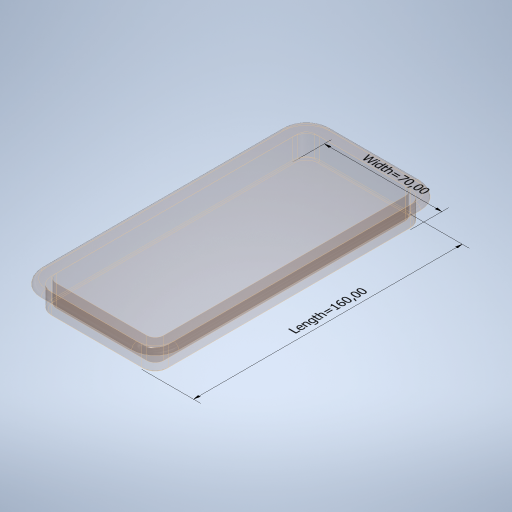
# Autodesk Inventor part: Holder for paper clips-01
Saved by Autodesk Inventor 2024 (Build 280153000, 153)
## iProperties
Company: UAB Čeli APS
Created: 2022-04-25
Part Number: Holder for paper clips-01
Material: Polycarbonate, Smoke
Document SubType Name: Modeling
Designer: sauliusd
Density: 1.2 g/cm^3
Appearance: Polycarbonate - Smoked
Description: Holder for paper clips.ipt
Width: 70,000 mm
Length: 160,000 mm
Author: S. Dereškevičius
Autodesk Inventor part; units mm, degrees
ref_plane "YZ Plane" through (0, 0, 0) normal (1, 0, 0) x (0, 1, 0)
ref_plane "XZ Plane" through (0, 0, 0) normal (0, 1, 0) x (-1, 0, 0)
ref_plane "XY Plane" through (0, 0, 0) normal (0, 0, 1) x (1, 0, 0)
sketch "Sketch1" plane through (0, 0, 0) normal (0, 0, 1) x (1, 0, 0)
  line L0 (-80, -35) -> (80, -35)
  line L1 (80, -35) -> (80, 35)
  line L2 (80, 35) -> (-80, 35)
  line L3 (-80, 35) -> (-80, -35)
  line L4 (-80, -35) -> (80, 35) construction
  line L5 (80, -35) -> (-80, 35) construction
  point P0 (0, 0)
  constraints: 12 end point, 2 midpoint, 2 parallel, 1 horizontal, 1 horizontal alignment, 1 perpendicular, 1 vertical alignment
extrude "Extrusion1" add sketch "Sketch1" along normal blind 13
fillet "Fillet1" radius 8 4 edges at (-80, -35, 6.5) (-80, 35, 6.5) (80, -35, 6.5) (80, 35, 6.5)
shell "Shell1" thickness 3 removed faces 1 at (24, -11.6667, 13)
sketch "Sketch2" plane through (0, 0, 13) normal (0, 0, 1) x (1, 0, 0)
  arc A0 (80, 27) -> (72, 35) centre (72, 27) ccw projected
  line L0 (72, 35) -> (-72, 35) projected
  arc A1 (-72, 35) -> (-80, 27) centre (-72, 27) ccw projected
  line L1 (-80, 27) -> (-80, -27) projected
  arc A2 (-80, -27) -> (-72, -35) centre (-72, -27) ccw projected
  line L2 (-72, -35) -> (72, -35) projected
  arc A3 (72, -35) -> (80, -27) centre (72, -27) ccw projected
  line L3 (80, -27) -> (80, 27) projected
  line L4 (-72, 41) -> (72, 41)
  arc A4 (86, 27) -> (72, 41) centre (72, 27) ccw
  line L5 (86, 27) -> (86, -27)
  arc A5 (72, -41) -> (86, -27) centre (72, -27) ccw
  line L6 (72, -41) -> (-72, -41)
  arc A6 (-86, -27) -> (-72, -41) centre (-72, -27) ccw
  line L7 (-86, -27) -> (-86, 27)
  arc A7 (-72, 41) -> (-86, 27) centre (-72, 27) ccw
  arc A8 (-72, 32) -> (-77, 27) centre (-72, 27) ccw projected
  line L8 (-72, 32) -> (72, 32) projected
  arc A9 (77, 27) -> (72, 32) centre (72, 27) ccw projected
  line L9 (77, 27) -> (77, -27) projected
  arc A10 (72, -32) -> (77, -27) centre (72, -27) ccw projected
  line L10 (72, -32) -> (-72, -32) projected
  arc A11 (-77, -27) -> (-72, -32) centre (-72, -27) ccw projected
  line L11 (-77, -27) -> (-77, 27) projected
  arc A12 (80, 27) -> (72, 35) centre (72, 27) ccw projected
  line L12 (72, 35) -> (-72, 35) projected
  arc A13 (-72, 35) -> (-80, 27) centre (-72, 27) ccw projected
  line L13 (-80, 27) -> (-80, -27) projected
  arc A14 (-80, -27) -> (-72, -35) centre (-72, -27) ccw projected
  line L14 (-72, -35) -> (72, -35) projected
  arc A15 (72, -35) -> (80, -27) centre (72, -27) ccw projected
  line L15 (80, -27) -> (80, 27) projected
  point P0 (0, 0)
  dimension "d5" = 6
  constraints: 8 end point, 8 point on circle, 4 centre point, 7 other
  measures "d5" distance between parallel lines of L0 L4
extrude "Extrusion2" add sketch "Sketch2" along normal blind 3 contours L3 A3 L2 A2 L1 A1 L0 A0 | L4 A4 L5 A5 L6 A6 L7 A7
fillet "Fillet2" radius 3 8 edges at (-86, 0, 16) (-81.8995, -36.8995, 16) (0, -41, 16) (81.8995, -36.8995, 16) (86, 0, 16) (81.8995, 36.8995, 16) (0, 41, 16) (-81.8995, 36.8995, 16)
sketch "Sketch3" plane through (0, 0, 0) normal (0, 0, -1) x (-1, 0, 0)
  arc A0 (-72, 35) -> (-80, 27) centre (-72, 27) ccw projected
  line L0 (-80, -27) -> (-80, 27) projected
  arc A1 (-80, -27) -> (-72, -35) centre (-72, -27) ccw projected
  line L1 (72, -35) -> (-72, -35) projected
  arc A2 (72, -35) -> (80, -27) centre (72, -27) ccw projected
  line L2 (80, 27) -> (80, -27) projected
  arc A3 (80, 27) -> (72, 35) centre (72, 27) ccw projected
  line L3 (-72, 35) -> (72, 35) projected
  point P0 (0, 0)
chamfer "Chamfer1" distance 1 angle 45 8 edges at (-80, 0, 0) (-77.6569, -32.6569, 0) (0, -35, 0) (77.6569, -32.6569, 0) (80, 0, 0) (77.6569, 32.6569, 0) (0, 35, 0) (-77.6569, 32.6569, 0)
extrude "Extrusion3" add sketch "Sketch3" against normal up to surface (13 mm away) separate body
sketch "Sketch4" plane through (-72, 35, 13) normal (0, 0, 1) x (1, 0, 0)
  line L0 (152, -8) -> (152, -62) projected
  line L1 (0, 0) -> (144, 0) projected
  point P0 (72, -35)
  point P1 (152, -35)
  point P2 (72, 0)
  constraints: 2 midpoint
equation "\"zzz\" = 1"
